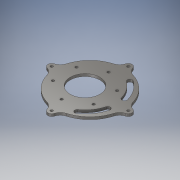
# Autodesk Inventor part: LargeBearingPlate
Saved by Autodesk Inventor 2019 (Build 230136000, 136)
## iProperties
Created: 2018-12-06
Part Number: LargeBearingPlate
Material: Stainless Steel
Document SubType Name: Modeling
Designer: steelen
Density: 8 g/cm^3
Appearance: Semi-Polished
Author: steelen
Autodesk Inventor part; units mm, degrees
ref_plane "YZ Plane" through (0, 0, 0) normal (1, 0, 0) x (0, 1, 0)
ref_plane "XZ Plane" through (0, 0, 0) normal (0, 1, 0) x (-1, 0, 0)
ref_plane "XY Plane" through (0, 0, 0) normal (0, 0, 1) x (1, 0, 0)
sketch "Sketch1" plane through (0, 0, 0) normal (0, 1, 0) x (-1, 0, 0)
  circle A0 centre (12.7, 0) radius 38.1
  circle A1 centre (0, 0) radius 88.9
  circle A2 centre (0, 98.425) radius 9.525
  arc A3 (9.1574, 101.0457) -> (24.7665, 85.3805) centre (31.1351, 107.3355) ccw
  arc A4 (-24.7665, 85.3805) -> (-9.1574, 101.0457) centre (-31.1351, 107.3355) ccw
  circle A5 centre (-98.425, 0) radius 9.525
  circle A6 centre (0, -98.425) radius 9.525
  circle A7 centre (98.425, 0) radius 9.525
  arc A8 (85.3805, 24.7665) -> (101.0457, 9.1574) centre (107.3355, 31.1351) ccw
  arc A9 (24.7665, -85.3805) -> (9.1574, -101.0457) centre (31.1351, -107.3355) ccw
  arc A10 (-9.1574, -101.0457) -> (-24.7665, -85.3805) centre (-31.1351, -107.3355) ccw
  arc A11 (-85.3805, -24.7665) -> (-101.0457, -9.1574) centre (-107.3355, -31.1351) ccw
  arc A12 (-101.0457, 9.1574) -> (-85.3805, 24.7665) centre (-107.3355, 31.1351) ccw
  arc A13 (101.0457, -9.1574) -> (85.3805, -24.7665) centre (107.3355, -31.1351) ccw
  line L0 (98.425, 0) -> (88.9, 0)
  line L1 (0, 98.425) -> (0, 88.9)
  line L2 (0, -98.425) -> (0, -88.9)
  line L3 (-98.425, 0) -> (-88.9, 0)
  line L4 (12.7, 0) -> (0, 0)
  dimension "d20" = 177.8
  dimension "d0" = 76.2
  dimension "d2" = 19.05
  dimension "d3" = 22.86
  dimension "d21" = 12.7
  constraints: 27 point on circle, 13 centre point, 10 end point, 10 equal radius, 8 tangent, 3 horizontal, 3 vertical, 1 coincident, 26 other
  measures "d0" diameter of A0
  measures "d2" diameter of A2
  measures "d3" radius of A10
  measures "d21" distance of L4.start point (0, 0)
extrude "Extrusion1" add sketch "Sketch1" along normal blind 6.35
sketch "Sketch3" plane through (0, 6.35, 0) normal (0, 1, 0) x (1, 0, 0)
  circle A0 centre (-12.7, 0) radius 38.1 projected
  arc A1 (101.0457, -9.1574) -> (101.0457, 9.1574) centre (98.425, 0) ccw projected
  arc A2 (101.0457, -9.1574) -> (85.3805, -24.7665) centre (107.3355, -31.1351) ccw projected
  arc A3 (24.7665, -85.3805) -> (85.3805, -24.7665) centre (0, 0) ccw projected
  arc A4 (24.7665, -85.3805) -> (9.1574, -101.0457) centre (31.1351, -107.3355) ccw projected
  arc A5 (-9.1574, -101.0457) -> (9.1574, -101.0457) centre (0, -98.425) ccw projected
  arc A6 (-9.1574, -101.0457) -> (-24.7665, -85.3805) centre (-31.1351, -107.3355) ccw projected
  arc A7 (-85.3805, -24.7665) -> (-24.7665, -85.3805) centre (0, 0) ccw projected
  arc A8 (-85.3805, -24.7665) -> (-101.0457, -9.1574) centre (-107.3355, -31.1351) ccw projected
  arc A9 (-101.0457, 9.1574) -> (-101.0457, -9.1574) centre (-98.425, 0) ccw projected
  arc A10 (-101.0457, 9.1574) -> (-85.3805, 24.7665) centre (-107.3355, 31.1351) ccw projected
  arc A11 (-24.7665, 85.3805) -> (-85.3805, 24.7665) centre (0, 0) ccw projected
  arc A12 (-24.7665, 85.3805) -> (-9.1574, 101.0457) centre (-31.1351, 107.3355) ccw projected
  arc A13 (9.1574, 101.0457) -> (-9.1574, 101.0457) centre (0, 98.425) ccw projected
  arc A14 (9.1574, 101.0457) -> (24.7665, 85.3805) centre (31.1351, 107.3355) ccw projected
  arc A15 (85.3805, 24.7665) -> (24.7665, 85.3805) centre (0, 0) ccw projected
  arc A16 (85.3805, 24.7665) -> (101.0457, 9.1574) centre (107.3355, 31.1351) ccw projected
  constraints: 4 coincident
hole "Hole1" at (98.425, 6.35, 0) at (0, 6.35, 98.425) at (-98.425, 6.35, 0) at (0, 6.35, -98.425) direction (0, -1, 0) diameter 6.5278 depth 12.2936 tip angle 118 clearance for "Socket Head Cap Screw" size "1/4" standard "Ansi Unified Screw Threads"
sketch "Sketch6" plane through (0, 0, 0) normal (0, -1, 0) x (1, 0, 0)
  circle A0 centre (-12.7, 0) radius 38.1 projected
  circle A1 centre (-12.7, 0) radius 50
  circle A2 centre (-12.7, 0) radius 69.85
  circle A3 centre (-12.7, 0) radius 60.325
  line L0 (-12.7, 0) -> (-12.7, 60.325)
  circle A4 centre (-12.7, 0) radius 60.325
  circle A5 centre (-12.7, 0) radius 60.325
  circle A6 centre (-12.7, 0) radius 60.325
  circle A7 centre (-12.7, 0) radius 60.325
  circle A8 centre (-12.7, 0) radius 60.325
  point P0 (0, 0)
  point P1 (39.543, 30.1625)
  point P2 (39.543, -30.1625)
  point P3 (-12.7, -60.325)
  point P4 (-64.943, -30.1625)
  point P5 (-64.943, 30.1625)
  dimension "d22" = 100
  dimension "d27" = 360
  dimension "d36" = 139.7
  dimension "d37" = 9.525
  constraints: 3 coincident, 2 centre point, 2 end point, 2 vertical alignment, 1 vertical, 35 other
  measures "d22" diameter of A1
  measures "d36" diameter of A2
hole "Hole2" at (-12.7, 0, 60.325) at (39.543, 0, 30.1625) at (39.543, 0, -30.1625) at (-12.7, 0, -60.325) at (-64.943, 0, -30.1625) at (-64.943, 0, 30.1625) direction (0, 1, 0) diameter 6.5278 depth 12.2936 tip angle 118 clearance for "Socket Head Cap Screw" size "1/4" standard "Ansi Unified Screw Threads"
sketch "Sketch8" plane through (0, 6.35, 0) normal (0, 1, 0) x (1, 0, 0)
  circle A0 centre (-12.7, 0) radius 38.1
  circle A1 centre (-12.7, 0) radius 76.2
  circle A2 centre (-12.7, 0) radius 88.9
  arc A3 (38.2909, 72.8226) -> (31.0065, 62.4194) centre (34.6487, 67.621) ccw
  arc A4 (31.0065, -62.4194) -> (38.2909, -72.8226) centre (34.6487, -67.621) ccw
  line L0 (2.6706, 21.8863) -> (60.2892, 21.8863)
  line L1 (-12.7, 0) -> (34.6487, 67.621)
  line L2 (34.6487, -67.621) -> (-12.7, 0)
  arc A5 (73.1708, -23.009) -> (60.9035, -19.722) centre (67.0372, -21.3655) ccw
  arc A6 (60.9035, 19.722) -> (73.1708, 23.009) centre (67.0372, 21.3655) ccw
  line L3 (-12.7, 0) -> (67.0372, 21.3655)
  line L4 (-12.7, 0) -> (67.0372, -21.3655)
  circle A7 centre (-12.7, 0) radius 38.1 projected
  point P0 (0, 0)
  dimension "d38" = 38.1
  dimension "d39" = 12.7
  dimension "d40" = 55
  dimension "d41" = 55
  dimension "d42" = 40
  dimension "d43" = 40
  constraints: 17 point on circle, 10 end point, 8 tangent, 7 centre point, 3 coincident, 2 concentric, 1 horizontal
  measures "d38" radial gap between concentric circles of A1 A0
  measures "d39" radial gap between concentric circles of A1 A2
  measures "d40" angle of L2 L0
  measures "d41" angle of L0 L1
  measures "d42" angle of L1 L3
  measures "d43" angle of L2 L4
extrude "Extrusion3" cut sketch "Sketch8" against normal blind 25.4 contours A1 A3 A2 A6 | A5 A2 A4 A1
body "Solid1"
